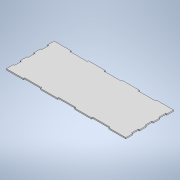
# Autodesk Inventor part: base
Saved by Autodesk Inventor 2020 (Build 240168000, 168)
## iProperties
Created: 2020-02-22
Part Number: base
Material: Generic
Document SubType Name: Modeling
Designer: udvarhelyi
Density: 1 g/cm^3
Appearance: Default
Author: udvarhelyi
Autodesk Inventor part; units mm, degrees
ref_plane "YZ Plane" through (0, 0, 0) normal (1, 0, 0) x (0, 1, 0)
ref_plane "XZ Plane" through (0, 0, 0) normal (0, 1, 0) x (-1, 0, 0)
ref_plane "XY Plane" through (0, 0, 0) normal (0, 0, 1) x (1, 0, 0)
sketch "Sketch1" plane through (0, 0, 0) normal (0, 1, 0) x (-1, 0, 0)
  line L0 (107.1429, 57) -> (107.1429, 60)
  line L1 (64.2857, 60) -> (64.2857, 57)
  line L2 (21.4286, 57) -> (21.4286, 60)
  line L3 (-21.4286, 60) -> (-21.4286, 57)
  line L4 (-64.2857, 60) -> (-64.2857, 57)
  line L5 (-107.1429, 57) -> (-107.1429, 60)
  line L6 (107.1429, -57) -> (107.1429, -60)
  line L7 (64.2857, -57) -> (64.2857, -60)
  line L8 (21.4286, -57) -> (21.4286, -60)
  line L9 (-21.4286, -57) -> (-21.4286, -60)
  line L10 (-64.2857, -57) -> (-64.2857, -60)
  line L11 (-107.1429, -57) -> (-107.1429, -60)
  line L12 (147, 25.7143) -> (150, 25.7143)
  line L13 (150, 8.5714) -> (147, 8.5714)
  line L14 (150, -8.5714) -> (147, -8.5714)
  line L15 (147, -25.7143) -> (150, -25.7143)
  line L16 (150, -42.8571) -> (147, -42.8571)
  line L17 (-147, -42.8571) -> (-150, -42.8571)
  line L18 (-150, -25.7143) -> (-147, -25.7143)
  line L19 (-147, 8.5714) -> (-150, 8.5714)
  line L20 (-147, 25.7143) -> (-150, 25.7143)
  line L21 (147, 42.8571) -> (150, 42.8571)
  line L22 (-150, -8.5714) -> (-147, -8.5714)
  line L23 (-147, 42.8571) -> (-150, 42.8571)
  line L24 (150, -42.8571) -> (150, -60)
  line L25 (147, -42.8571) -> (147, -25.7143)
  line L26 (150, -8.5714) -> (150, -25.7143)
  line L27 (147, -8.5714) -> (147, 8.5714)
  line L28 (147, 25.7143) -> (147, 42.8571)
  line L29 (150, 60) -> (150, 42.8571)
  line L30 (150, 25.7143) -> (150, 8.5714)
  line L31 (107.1429, 60) -> (150, 60)
  line L32 (107.1429, 57) -> (64.2857, 57)
  line L33 (150, -60) -> (107.1429, -60)
  line L34 (64.2857, -60) -> (21.4286, -60)
  line L35 (-21.4286, -60) -> (-64.2857, -60)
  line L36 (-107.1429, -60) -> (-150, -60)
  line L37 (64.2857, -57) -> (107.1429, -57)
  line L38 (-107.1429, -57) -> (-64.2857, -57)
  line L39 (-21.4286, -57) -> (21.4286, -57)
  line L40 (21.4286, 60) -> (64.2857, 60)
  line L41 (21.4286, 57) -> (-21.4286, 57)
  line L42 (-64.2857, 57) -> (-107.1429, 57)
  line L43 (-150, 60) -> (-107.1429, 60)
  line L44 (-64.2857, 60) -> (-21.4286, 60)
  line L45 (-147, -25.7143) -> (-147, -42.8571)
  line L46 (-147, 42.8571) -> (-147, 25.7143)
  line L47 (-147, 8.5714) -> (-147, -8.5714)
  line L48 (-150, 42.8571) -> (-150, 60)
  line L49 (-150, 8.5714) -> (-150, 25.7143)
  line L50 (-150, -60) -> (-150, -42.8571)
  line L51 (-150, -25.7143) -> (-150, -8.5714)
  point P0 (0, 0)
  dimension "d6" = 85.7143
  dimension "d17" = 17.1429
  dimension "d18" = 34.2857
  dimension "d19" = 51.4286
  dimension "d20" = 68.5714
  dimension "d21" = 85.7143
  dimension "d22" = 102.8571
  dimension "d23" = 120
  dimension "d24" = 150
  dimension "d25" = 300
  dimension "d26" = 42.8571
  dimension "d27" = 128.5714
  dimension "d28" = 171.4286
  dimension "d29" = 214.2857
  dimension "d30" = 257.1429
  dimension "d34" = 3
  dimension "d35" = 3
  dimension "d36" = 60
  dimension "d37" = 3
  dimension "d38" = 3
  constraints: 104 end point, 93 perpendicular, 51 parallel, 28 collinear, 8 point on line, 4 horizontal
  measures "d6" horizontal distance of L29.start L1.end
  measures "d17" distance from line of L16.start L33
  measures "d18" distance from line of L33 L15.end
  measures "d19" distance from line of L14.start L33
  measures "d20" distance from line of L13.start L33
  measures "d21" distance from line of L12.start L33
  measures "d22" distance from line of L21.end L33
  measures "d23" distance between parallel lines of L31 L33
  measures "d24" distance from line of point (0, 0) L24
  measures "d25" distance from line of L36.end L24
  measures "d26" distance from line of L0.end L29
  measures "d27" distance from line of L2.start L29
  measures "d28" distance from line of L3.start L29
  measures "d29" distance from line of L4.end L29
  measures "d30" distance from line of L29 L5.end
  measures "d34" distance between parallel lines of L50 L45
  measures "d35" distance of L11.start L11.end
  measures "d36" distance from line of L35 point (0, 0)
  measures "d37" distance of L0.start L0.end
  measures "d38" distance of L21.start L21.end
extrude "Extrusion1" add sketch "Sketch1" along normal blind 3
equation "\"d6\" = 0.285714 * wt - tol"
equation "\"d17\" = d11"
equation "\"d18\" = d12"
equation "\"d19\" = d13"
equation "\"d20\" = d14"
equation "\"d21\" = d15"
equation "\"d22\" = d16"
equation "\"d23\" = ht"
equation "\"d24\" = 0.5 * wt"
equation "\"d25\" = wt"
equation "\"d26\" = d5"
equation "\"d27\" = d7"
equation "\"d28\" = d8"
equation "\"d29\" = d9"
equation "\"d30\" = d10"
equation "\"d34\" = tt"
equation "\"d35\" = tt"
equation "\"d36\" = 0.5 * ht"
equation "\"d37\" = tt"
equation "\"d38\" = tt"
equation "\"d31\" = tt"
equation "\"d4\" = tt"
equation "\"wt\" = 300"
equation "\"ht\" = 120"
equation "\"tt\" = 3"
equation "\"tol\" = 0"
equation "\"d5\" = 0.142857 * wt + tol"
equation "\"d7\" = 0.428571 * wt + tol"
equation "\"d8\" = 0.571429 * wt - tol"
equation "\"d9\" = 0.714286 * wt + tol"
equation "\"d10\" = 0.857143 * wt - tol"
equation "\"d11\" = 0.142857 * ht + tol"
equation "\"d12\" = 0.285714 * ht - tol"
equation "\"d13\" = 0.428571 * ht + tol"
equation "\"d14\" = 0.571429 * ht - tol"
equation "\"d15\" = 0.714286 * ht + tol"
equation "\"d16\" = 0.857143 * ht - tol"
equation "\"tiroir\" = 1"
equation "\"nHoles\" = 4"
equation "\"shelfH\" = 35"
body "Solid1"
